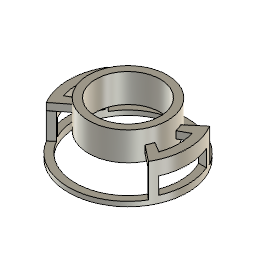
音响holder (Autodesk Fusion 360 design; units mm, degrees)
part number: 2025-11-05-10-08-59-068
Autodesk Fusion 360 part; units mm, degrees
note: some values were not read from the file. Set by a fixed rule: which face or edge a step refers to.
sketch "Sketch1" plane through (0, 0, 0) normal (0, 0, 1) x (1, 0, 0)
  circle A0 centre (0, 0) radius 22
  circle A1 centre (0, 0) radius 25
  dimension "d1" = 44
  dimension "d2" = 50
  constraint coincident A0.centre A1.centre
  constraint concentric A0 A1
  measures "d1" diameter of A0
  measures "d2" diameter of A1
extrude "Extrude1" add sketch "Sketch1" along normal blind 2 makes body 1
sketch "Sketch2" plane through (0, 0, 2) normal (0, 0, 1) x (-1, 0, 0)
  circle A0 centre (0, 0) radius 22
  circle A1 centre (0, 0) radius 25
  circle A2 centre (0, 0) radius 22
  circle A3 centre (0, 0) radius 25
  line L0 (21.4312, -12.8726) -> (19.1226, -10.8777)
  line L1 (21.4312, 12.8726) -> (19.1226, 10.8777)
  line L2 (-21.4312, -12.8726) -> (-19.1226, -10.8777)
  line L3 (-21.4312, 12.8726) -> (-19.1226, 10.8777)
  constraint concentric A0 A2
  constraint concentric A2 A3
  constraint coincident A3 L0.start
  constraint coincident A0 L0.end
  constraint coincident A1 L1.start
  constraint coincident A2 L1.end
  constraint coincident A1 L2.start
  constraint coincident A0 L2.end
  constraint parallel L1 L2
  constraint coincident A3 L3.start
  constraint coincident A2 L3.end
  constraint parallel L0 L3
extrude "Extrude2" add sketch "Sketch2" along normal blind 15 contours A0 A1 A2 A3 L0 L1 | A0 A1 A2 A3 L2 L3 bodies 1
sketch "Sketch3" plane through (0, 0, 17) normal (0, 0, 1) x (-1, 0, 0)
  arc A0 (21.4312, -12.8726) -> (21.4312, 12.8726) centre (0, 0) ccw
  line L0 (21.4312, 12.8726) -> (19.1226, 10.8777)
  arc A1 (19.1226, -10.8777) -> (19.1226, 10.8777) centre (0, 0) ccw
  line L1 (19.1226, -10.8777) -> (21.4312, -12.8726)
  circle A2 centre (0, 0) radius 13.5
  circle A3 centre (0, 0) radius 16.5695
  dimension "d7" = 27
  constraint concentric A0 A2
  constraint concentric A2 A3
  measures "d7" diameter of A2
extrude "Extrude3" add sketch "Sketch3" along normal blind 5 separate body contours A3 makes body 2
extrude "Extrude4" add 2 faces at (-23.9039, -1.6648, 17) (23.9039, 1.6648, 17) along direction (0, 0, 1) blind 5 on bodies 1 bodies 1
extrude "Extrude5" add 1 faces at (-15.4344, 1.4939, 17) along direction (0, 0, -1) blind 7 on bodies 2 bodies 2
extrude "Extrude6" cut 2 faces at (-23.9039, -1.6648, 22) (23.9039, 1.6648, 22) along direction (0, 0, -1) blind 6 on bodies 1 bodies 1
sketch "Sketch4" plane through (0, 0, 16) normal (0, 0, 1) x (-1, 0, 0)
  arc A0 (21.4312, -12.8726) -> (21.4312, 12.8726) centre (0, 0) ccw
  line L0 (21.4312, 12.8726) -> (19.1226, 10.8777)
  arc A1 (19.1226, -10.8777) -> (19.1226, 10.8777) centre (0, 0) ccw
  line L1 (19.1226, -10.8777) -> (21.4312, -12.8726)
  line L2 (21.4312, 12.8726) -> (14, 7)
  line L3 (14, 7) -> (14, -6.4511)
  line L4 (14, -6.4511) -> (21.4312, -12.8726)
  constraint coincident A0.end L0.start
  constraint vertical L3
  constraint coincident A0.start L1.end
  constraint parallel L1 L4
extrude "Extrude7" add sketch "Sketch4" against normal blind 3 contours L0 A1 L2 L3 L4 bodies 1 2
mirror "Mirror1" about plane through (0, 0, 0) normal (1, 0, 0) of "Extrude7"
sketch "Sketch5" plane through (0, 0, 0) normal (1, 0, 0) x (0, 1, 0)
  line L0 (-10, 10) -> (10, 10)
  line L1 (10, 10) -> (10, 3)
  line L2 (10, 3) -> (-10, 3)
  line L3 (-10, 3) -> (-10, 10)
  constraint horizontal L0
  constraint vertical L1
  constraint horizontal L2
  constraint vertical L3
extrude "Extrude8" cut sketch "Sketch5" along normal mid plane 54 bodies 1
sketch "Sketch6" plane through (0, 0, 16) normal (0, 0, 1) x (-1, 0, 0)
  arc A0 (21.4312, -12.8726) -> (21.4312, 12.8726) centre (0, 0) ccw
  line L0 (21.4312, 12.8726) -> (14.734, 7.5801)
  arc A1 (14.9067, -7.2346) -> (14.734, 7.5801) centre (0, 0) ccw
  line L1 (14.9067, -7.2346) -> (21.4312, -12.8726)
  circle A2 centre (0, 0) radius 16.5695
  circle A3 centre (0, 0) radius 21.3776
  line L2 (-20.1345, 7.1834) -> (-15.9102, 4.6275)
  line L3 (-20.3781, -6.4601) -> (-16.05, -4.1167)
  line L4 (15.9696, 4.4183) -> (20.2828, 6.7535)
  line L5 (16.1229, -3.8213) -> (20.3951, -6.4063)
  constraint concentric A0 A2
  constraint concentric A2 A3
  constraint coincident A3 L2.start
  constraint coincident A2 L2.end
  constraint coincident A3 L3.start
  constraint coincident A2 L3.end
  constraint coincident A1 L4.start
  constraint coincident A2 L4.start
  constraint coincident A3 L4.end
  constraint parallel L3 L4
  constraint coincident A1 L5.start
  constraint coincident A3 L5.end
  constraint parallel L2 L5
extrude "Extrude9" cut sketch "Sketch6" against normal blind 8 contours A2 A3 L2 L3 | A1 A2 A3 L4 L5 bodies 1
